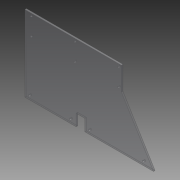
# Autodesk Inventor part: Hopper Left Side Leg
Saved by Autodesk Inventor 2014 SP1 (Build 180222100, 222)
## iProperties
Created: 2013-12-16
Part Number: Hopper Left Side Leg
Material: Polycarbonate, Clear
Document SubType Name: Modeling
Designer: Moses
Mass: 144.824 g
Surface Area: 791.898 cm^2
Volume: 120.687 cm^3
Density: 1.2 g/cm^3
Appearance: Polycarbonate - Clear
Author: Moses
Autodesk Inventor part; units mm, degrees
ref_plane "YZ Plane" through (0, 0, 0) normal (1, 0, 0) x (0, 1, 0)
ref_plane "XZ Plane" through (0, 0, 0) normal (0, 1, 0) x (-1, 0, 0)
ref_plane "XY Plane" through (0, 0, 0) normal (0, 0, 1) x (1, 0, 0)
sketch "Sketch1" plane through (0, 0, 0) normal (0, 0, 1) x (1, 0, 0)
  line L0 (0, 0) -> (279.4, 0)
  line L1 (0, 0) -> (0, 165.1)
  line L2 (0, 165.1) -> (209.55, 165.1)
  line L3 (209.55, 165.1) -> (209.55, 114.3)
  line L4 (209.55, 114.3) -> (279.4, 0)
  circle A0 centre (9.525, 7.9375) radius 1.905 projected
  circle A1 centre (98.425, 7.9375) radius 1.905 projected
  line L5 (111.125, 0) -> (111.125, 25.4)
  line L6 (111.125, 25.4) -> (130.175, 25.4)
  line L7 (130.175, 25.4) -> (130.175, 0)
  circle A2 centre (12.7, 158.75) radius 1.5875
  circle A3 centre (107.95, 158.75) radius 1.5875
  circle A4 centre (203.2, 158.75) radius 1.5875
  circle A5 centre (12.7, 120.65) radius 1.5875
  circle A6 centre (107.95, 120.65) radius 1.5875
  circle A7 centre (203.2, 120.65) radius 1.5875
  circle A8 centre (139.7, 7.9375) radius 1.905 projected
  circle A9 centre (257.175, 7.9375) radius 1.905 projected
  line L8 (133.35, 0) -> (133.35, 15.875) construction
  line L9 (133.35, 0) -> (266.7, 0) construction
  line L10 (266.7, 15.875) -> (266.7, 0) construction
  line L11 (133.35, 15.875) -> (266.7, 15.875) construction
  dimension "d0" = 279.4
  dimension "d1" = 165.1
  dimension "d2" = 209.55
  dimension "d3" = 50.8
  dimension "d6" = 19.05
  dimension "d7" = 25.4
  dimension "d8" = 12.7
  dimension "d9" = 3.175
  dimension "d12" = 95.25
  dimension "d15" = 38.1
  dimension "d18" = 12.7
  dimension "d19" = 6.35
  constraints: 16 end point, 6 centre point, 3 horizontal, 3 vertical, 2 perpendicular, 2 point on line, 1 coincident, 1 parallel, 10 other
  measures "d0" distance of L0.start L0.end
  measures "d1" distance of L0.start L1.end
  measures "d2" distance of L1.end L2.end
  measures "d3" distance of L2.end L3.end
  measures "d6" distance of L5.end L6.end
  measures "d7" distance of L5.start L5.end
  measures "d8" distance from line of A1.centre L5
  measures "d9" diameter of A2
  measures "d12" distance of A2.centre A3.centre
  measures "d15" distance of A2.centre A5.centre
  measures "d18" distance from line of A2.centre L1
  measures "d19" distance from line of L2 A2.centre
extrude "Extrusion1" add sketch "Sketch1" along normal blind 3.175 contours L1 L2 L3 L4 L0 L7 L6 L5
body "Solid1"
